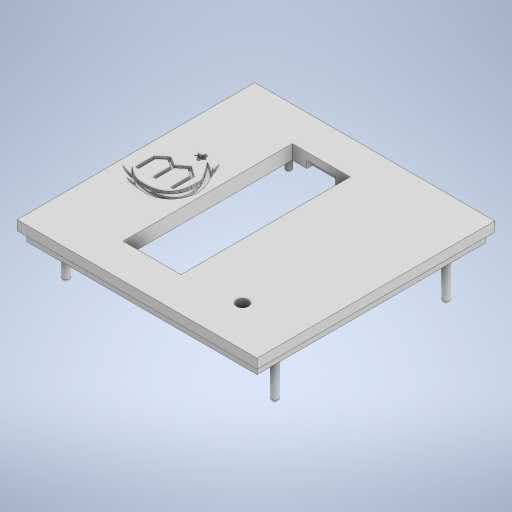
# Autodesk Inventor part: base_frontal_esp
Saved by Autodesk Inventor 2023 (Build 270158000, 158)
## iProperties
Created: 2022-11-29
Part Number: base_frontal_esp
Material: Genérico
Document SubType Name: Modeling
Designer: Inteli
Density: 1 g/cm^3
Appearance: Padrão
Author: Inteli
## iProperties of the stored document base_frontal_esp_3DPrint.ipt
Created: 2022-11-29
Part Number: base_frontal_esp_3DPrint
Material: Genérico
Document SubType Name: Modeling
Designer: Inteli
Density: 1 g/cm^3
Appearance: Padrão
Author: Inteli
Autodesk Inventor part; units mm, degrees
ref_plane "YZ Plane" through (0, 0, 0) normal (1, 0, 0) x (0, 1, 0)
ref_plane "XZ Plane" through (0, 0, 0) normal (0, 1, 0) x (-1, 0, 0)
ref_plane "XY Plane" through (0, 0, 0) normal (0, 0, 1) x (1, 0, 0)
sketch "Esboço1" plane through (0, 0, 0) normal (0, 1, 0) x (-1, 0, 0)
  line L0 (50.5, 50) -> (-50.5, 50)
  line L1 (-50.5, 50) -> (-50.5, -50)
  line L2 (-50.5, -50) -> (50.5, -50)
  line L3 (50.5, -50) -> (50.5, 50)
  line L4 (50.5, 50) -> (-50.5, -50) construction
  line L5 (-50.5, 50) -> (50.5, -50) construction
  line L6 (20.2995, 35.575) -> (-4.0005, 35.575)
  line L7 (-4.0005, 35.575) -> (-4.0005, -35.575)
  line L8 (-4.0005, -35.575) -> (20.2995, -35.575)
  line L9 (20.2995, -35.575) -> (20.2995, 35.575)
  line L10 (20.2995, 35.575) -> (-4.0005, -35.575) construction
  line L11 (-4.0005, 35.575) -> (20.2995, -35.575) construction
  line L12 (44.809, 5.8351) -> (43.5847, 5.8351)
  line L13 (43.5847, 5.8351) -> (43.5847, -1.2807)
  line L14 (44.809, -1.7713) -> (44.809, 5.8351)
  line L15 (37.4674, -1.5814) -> (37.4674, 5.8351)
  line L16 (36.2814, 5.8351) -> (36.3184, -1.9609)
  line L17 (37.4674, 5.8351) -> (36.2814, 5.8351)
  arc A0 (45.6383, 6.4318) -> (42.5276, 9.5405) centre (27.0068, -9.1007) ccw
  arc A1 (45.6383, 6.4318) -> (40.7813, 9.7169) centre (35.3189, -3.5922) ccw
  arc A2 (48.2046, 8.0198) -> (42.5276, 9.5405) centre (39.1563, -14.4019) ccw
  arc A3 (48.2046, 8.0198) -> (40.2854, 11.1296) centre (34.1591, -16.1096) ccw
  arc A4 (40.7813, 9.7169) -> (36.9942, 10.6964) centre (35.3189, -3.5922) ccw
  arc A5 (42.5276, 9.5405) -> (40.2854, 11.1296) centre (31.511, -3.6276) ccw
  arc A6 (42.5276, 9.5405) -> (39.5218, 11.5577) centre (31.511, -3.6276) ccw
  arc A7 (42.6579, 11.5577) -> (38.6679, 12.02) centre (38.9758, -2.7706) ccw
  arc A8 (42.6579, 11.5577) -> (39.3141, 12.7524) centre (36.6829, 0.1114) ccw
  arc A9 (39.5218, 11.5577) -> (37.8822, 12.3788) centre (32.6692, -0.0774) ccw
  arc A10 (32.6917, 13.3458) -> (28.802, 12.3788) centre (32.9881, 3.847) ccw
  arc A11 (32.9881, 10.9892) -> (31.7772, 10.4136) centre (38.1916, -1.5183) ccw
  arc A12 (28.802, 12.3788) -> (27.4641, 11.6847) centre (32.6917, 3.2455) ccw
  arc A13 (31.7772, 10.4136) -> (30.4336, 9.6603) centre (40.3851, -6.5145) ccw
  arc A14 (32.6139, 10.9611) -> (29.2079, 10.2542) centre (33.9158, -3.8703) ccw
  arc A15 (32.8836, 9.8314) -> (30.7097, 9.0348) centre (35.8636, -1.665) ccw
  arc A16 (27.4641, 11.6847) -> (26.2813, 10.8254) centre (32.6917, 3.2455) ccw
  arc A17 (29.2079, 10.2542) -> (27.3406, 9.3519) centre (31.9412, 2.2141) ccw
  arc A18 (29.5501, 9.0348) -> (28.6058, 8.2482) centre (39.1969, -3.5073) ccw
  arc A19 (26.2813, 10.8254) -> (24.8245, 9.2999) centre (32.6917, 3.2455) ccw
  arc A20 (30.7097, 9.0348) -> (29.0216, 7.805) centre (34.0907, 2.6203) ccw
  arc A21 (27.3406, 9.3519) -> (25.7439, 8.0198) centre (31.9412, 2.2141) ccw
  arc A22 (28.6058, 8.2482) -> (27.662, 7.2379) centre (33.3062, 2.9113) ccw
  arc A23 (24.8245, 9.2999) -> (23.5927, 7.4677) centre (38.9166, -1.505) ccw
  arc A24 (30.4336, 9.6603) -> (29.5501, 9.0348) centre (32.8777, 5.2714) ccw
  arc A25 (24.7648, 6.4318) -> (24.4302, 5.4014) centre (28.6882, 4.5883) ccw
  arc A26 (25.7439, 8.0198) -> (24.7648, 6.4318) centre (32.6186, 2.6854) ccw
  arc A27 (23.5927, 7.4677) -> (22.4449, 3.8607) centre (35.0612, 1.8321) ccw
  arc A28 (26.6056, 5.7739) -> (25.8372, 4.2176) centre (36.8949, -0.274) ccw
  arc A29 (25.8372, 4.2176) -> (25.1763, 1.9892) centre (36.8949, -0.274) ccw
  arc A30 (24.4302, 5.4014) -> (24.3636, 1.8425) centre (33.2592, 3.4561) ccw
  arc A31 (27.0068, 4.8466) -> (26.3681, 2.5448) centre (34.7317, 1.4636) ccw
  arc A32 (22.4449, 3.8607) -> (22.3296, 1.6755) centre (31.1835, 2.304) ccw
  arc A33 (26.3681, 2.5448) -> (26.168, 1.1642) centre (413.7374, -54.3143) ccw
  line L18 (29.975, 5.8351) -> (28.8297, 5.8351)
  arc A34 (22.3296, 1.6755) -> (23.1987, -2.3386) centre (36.0492, 2.5448) ccw
  arc A35 (25.1763, 1.9892) -> (24.9935, -0.598) centre (35.3122, -0.0273) ccw
  arc A36 (26.168, 1.1642) -> (26.0888, -0.901) centre (41.6964, -0.4656) ccw
  arc A37 (24.3636, 1.8425) -> (25.65, -2.2141) centre (40.1319, 4.6107) ccw
  arc A38 (26.0888, -0.901) -> (26.168, -3.3028) centre (40.7425, -1.6198) ccw
  line L19 (28.8297, 5.8351) -> (28.8297, -2.8363)
  line L20 (29.975, -2.2568) -> (29.975, 5.8351)
  line L21 (33.2053, -4.5224) -> (29.975, -2.2568)
  line L22 (28.8297, -2.8363) -> (33.2418, -6.0041)
  line L23 (36.3184, -1.9609) -> (33.2053, -4.5224)
  line L24 (40.8957, -3.6276) -> (37.4674, -1.5814)
  line L25 (33.2418, -6.0041) -> (37.1716, -2.7706)
  line L26 (37.1716, -2.7706) -> (41.0273, -5.0718)
  arc A39 (27.662, 7.2379) -> (26.6056, 5.7739) centre (37.4265, -0.9211) ccw
  arc A40 (29.0216, 7.805) -> (27.0068, 4.8466) centre (34.5802, 1.8542) ccw
  arc A41 (25.65, -2.2141) -> (27.7622, -5.9921) centre (47.4025, 7.4677) ccw
  arc A42 (24.9935, -5.6255) -> (26.0942, -6.9357) centre (36.0492, 2.5448) ccw
  arc A43 (24.9935, -5.6255) -> (25.4758, -7.1596) centre (38.388, -2.2568) ccw
  arc A44 (24.4302, -4.8024) -> (26.8873, -7.7042) centre (36.0492, 2.5448) ccw
  arc A45 (23.1987, -2.3386) -> (24.4302, -4.8024) centre (36.0492, 2.5448) ccw
  line L27 (43.5847, -1.2807) -> (40.8957, -3.6276)
  line L28 (41.0273, -5.0718) -> (44.809, -1.7713)
  line L29 (34.2937, -11.1823) -> (34.0945, -11.0661)
  line L30 (33.8991, -11.0325) -> (33.7636, -10.9072)
  line L31 (33.3989, -11.5321) -> (33.7389, -12.1961)
  line L32 (33.7389, -12.1961) -> (33.9199, -12.0962)
  line L33 (33.5923, -12.4562) -> (34.3671, -12.0313)
  line L34 (33.9199, -12.0962) -> (33.608, -11.5313)
  line L35 (33.5136, -10.9851) -> (32.8806, -11.5321)
  line L36 (33.6313, -10.6456) -> (32.6918, -11.5321)
  line L37 (33.1875, -11.5438) -> (33.5136, -10.9851)
  line L38 (33.8225, -11.5321) -> (34.0691, -12.0138)
  line L39 (34.0691, -12.0138) -> (34.2937, -11.8898)
  line L40 (33.7636, -10.9072) -> (33.3989, -11.5321)
  line L41 (33.608, -11.5313) -> (33.8991, -11.0325)
  line L42 (34.0945, -11.0661) -> (33.8225, -11.5321)
  line L43 (34.3671, -11.0482) -> (33.6313, -10.6456)
  line L44 (33.5136, -10.0703) -> (34.3671, -11.0482)
  line L45 (34.2937, -11.1823) -> (34.2937, -11.8898)
  line L46 (32.8806, -11.5321) -> (33.4944, -12.0996)
  line L47 (32.6918, -11.5321) -> (33.5923, -12.4562)
  line L48 (33.4944, -12.0996) -> (33.1875, -11.5438)
  arc A46 (25.4758, -7.1596) -> (26.168, -8.8375) centre (37.6572, -3.116) ccw
  arc A47 (26.0942, -6.9357) -> (27.0629, -8.5615) centre (38.5577, -0.6105) ccw
  arc A48 (27.0629, -8.5615) -> (27.4344, -9.9972) centre (63.4878, 0.0976) ccw
  arc A49 (27.0629, -8.5615) -> (28.2466, -10.17) centre (40.1173, -0.1951) ccw
  arc A50 (26.8873, -7.7042) -> (28.2466, -10.17) centre (61.1895, 9.5979) ccw
  arc A51 (27.4344, -9.9972) -> (27.7155, -11.1094) centre (75.5076, 1.5619) ccw
  arc A52 (26.8687, -10.2938) -> (27.4238, -11.3917) centre (91.8054, 21.8477) ccw
  arc A53 (27.7622, -5.9921) -> (31.3672, -10.9259) centre (68.3902, 19.9095) ccw
  arc A54 (26.8873, -7.7042) -> (31.3672, -10.9259) centre (41.3631, 7.6994) ccw
  arc A55 (27.7155, -11.1094) -> (28.1199, -12.5465) centre (75.5076, 1.5619) ccw
  arc A56 (27.4238, -11.3917) -> (28.1199, -12.5465) centre (38.8613, -5.2849) ccw
  arc A57 (26.168, -8.8375) -> (26.8687, -10.2938) centre (91.8054, 21.8477) ccw
  line L49 (34.8442, -10.3512) -> (34.6787, -9.7074)
  line L50 (34.6787, -9.7074) -> (33.9642, -9.5676)
  line L51 (34.8442, -10.8775) -> (34.8442, -10.3512)
  line L52 (33.9642, -9.5676) -> (33.5136, -10.0703)
  line L53 (34.6829, -11.4101) -> (34.8442, -10.8775)
  line L54 (34.3671, -11.0482) -> (34.6829, -11.4101)
  line L55 (34.6829, -11.6897) -> (34.8442, -12.2373)
  line L56 (34.3671, -12.0313) -> (34.6829, -11.6897)
  line L57 (34.8442, -12.2373) -> (35.1652, -12.4348)
  arc A58 (39.9353, 10.0335) -> (35.0612, 10.1842) centre (36.8756, -10.0261) ccw
  arc A59 (35.0612, 10.1842) -> (32.8836, 9.8314) centre (35.8636, -1.665) ccw
  arc A60 (36.9942, 10.6964) -> (32.6139, 10.9611) centre (33.9158, -3.8703) ccw
  arc A61 (37.8822, 12.3788) -> (35.3189, 13.1632) centre (32.6692, -0.0774) ccw
  arc A62 (35.3189, 13.1632) -> (32.6917, 13.3458) centre (33.3374, 3.6492) ccw
  arc A63 (39.3141, 12.7524) -> (34.7317, 13.2668) centre (35.1345, -3.8139) ccw
  line L58 (34.8798, -12.783) -> (34.8442, -12.2373)
  line L59 (34.3671, -12.0313) -> (33.4944, -12.975)
  line L60 (33.9307, -13.475) -> (34.6371, -13.3962)
  line L61 (33.4944, -12.975) -> (33.9307, -13.475)
  line L62 (34.6371, -13.3962) -> (34.8798, -12.783)
  line L63 (35.1652, -12.4348) -> (35.9116, -11.9781)
  line L64 (35.1345, -10.6456) -> (34.8442, -10.8775)
  arc A64 (36.566, -12.5465) -> (36.62, -12.3703) centre (36.3795, -12.3929) ccw
  arc A65 (36.566, -12.5465) -> (35.9116, -11.8619) centre (35.6269, -12.789) ccw
  line L65 (35.9116, -11.9781) -> (35.9116, -11.1094)
  arc A66 (36.62, -12.3703) -> (35.9116, -11.6487) centre (35.5381, -12.7239) ccw
  line L66 (35.9116, -11.1094) -> (35.1345, -10.6456)
  arc A67 (35.9116, -11.3917) -> (36.62, -10.6875) centre (35.6092, -10.3791) ccw
  arc A68 (35.9116, -11.2016) -> (36.5905, -10.5013) centre (35.3642, -9.9917) ccw
  arc A69 (36.62, -10.6875) -> (36.5905, -10.5013) centre (36.2493, -10.6509) ccw
  point P0 (0, 0)
  point P1 (28.6058, 8.2482)
  dimension "d0" = 101
  dimension "d1" = 100
  dimension "d2" = 24.3
  dimension "d3" = 71.15
  constraints: 165 point on circle, 134 end point, 70 centre point, 16 parallel, 12 point on line, 10 concentric, 8 perpendicular, 3 horizontal, 3 vertical, 2 midpoint
  measures "d0" distance of L2.end L1.end
  measures "d1" distance of L1.end L0.end
  measures "d2" distance of L8.end L7.end
  measures "d3" distance of L7.end L6.end
extrude "Base" add sketch "Esboço1" against normal blind 8 contours L3 L2 L1 L0 | L14 L28 L26 L25 L22 L19 L18 L20 L21 L23 L16 L17 L15 L24 L27 L13 L12 | A1 A4 A60 A14 A17 A21 A26 A25 A30 A37 A41 A53 A54 A44 A42 A45 A34 A32 A27 A23 A19 A16 A12 A10 A62 A61 A9 A6 A5 A0 | A5 A3 A2 | A58 A59 A15 A20 A40 A31 A33 A36 A38 A41 A37 A35 A29 A28 A39 A22 A18 A24 A13 A11 A60 A4 | A9 A61 A62 A63 A8 A7 | A11 A13 A24 A18 A22 A39 A28 A29 A35 A37 A30 A25 A26 A21 A17 A14 A60 | A50 A49 A47 A44 | A47 A48 A51 A55 A56 A52 A57 A46 A43 A42 | L45 L39 L38 L42 L29 | L41 L34 L32 L31 L40 L30 | L47 L36 L43 L54 L53 L64 L66 L65 L63 L57 L55 L56 L33 | L56 L55 L58 L62 L60 L61 L59 | L44 L52 L50 L49 L51 L53 L54 | L65 A66 A64 A65 | L65 A68 A69 A67 | L37 L48 L46 L35
sketch "Esboço4" plane through (0, -8, 0) normal (0, -1, 0) x (1, 0, 0)
  line L0 (-48, 40) -> (-48, -40) projected
  line L1 (48, -40) -> (48, 40) projected
  circle A0 centre (-44, -36) radius 1.5
  circle A1 centre (-44, 36) radius 1.5
  circle A2 centre (44, 36) radius 1.5
  circle A3 centre (44, -36) radius 1.5
  line L2 (-50.5, 50) -> (-50.5, -50) projected
  line L3 (50.5, 50) -> (-50.5, 50) projected
  point P0 (0, 0)
  dimension "d21" = 3
  dimension "d22" = 3
  dimension "d23" = 3
  dimension "d24" = 3
  dimension "d82" = 6.5
  dimension "d83" = 14
  constraints: 4 centre point
  measures "d21" diameter of A0
  measures "d22" diameter of A1
  measures "d23" diameter of A2
  measures "d24" diameter of A3
  measures "d82" distance from line of L2 A1.centre
  measures "d83" distance from line of L3 A1.centre
extrude "Pinos_encaixe" add sketch "Esboço4" along normal blind 18
fillet "Arredondamento_pino" radius 1.5 4 edges at (-45.5, -26, -36) (-45.5, -26, 36) (42.5, -26, 36) (42.5, -26, -36)
extrude "Logo Iobee C.1" cut sketch "Esboço1" against normal blind 1.5 contours L14 L28 L26 L25 L22 L19 L18 L20 L21 L23 L16 L17 L15 L24 L27 L13 L12 | A1 A4 A60 A14 A17 A21 A26 A25 A30 A37 A41 A53 A54 A44 A42 A45 A34 A32 A27 A23 A19 A16 A12 A10 A62 A61 A9 A6 A5 A0 | L45 L39 L38 L42 L29 | L41 L34 L32 L31 L40 L30 | L47 L36 L43 L54 L53 L64 L66 L65 L63 L57 L55 L56 L33 | L56 L55 L58 L62 L60 L61 L59 | L44 L52 L50 L49 L51 L53 L54 | L65 A66 A64 A65 | L65 A68 A69 A67 | L37 L48 L46 L35
extrude "Logo Iobee C.2" cut sketch "Esboço1" against normal blind 1 contours A5 A3 A2 | A58 A59 A15 A20 A40 A31 A33 A36 A38 A41 A37 A35 A29 A28 A39 A22 A18 A24 A13 A11 A60 A4 | A47 A48 A51 A55 A56 A52 A57 A46 A43 A42
extrude "Logo Iobee C.3" cut sketch "Esboço1" against normal blind 0.5 contours A9 A61 A62 A63 A8 A7 | A11 A13 A24 A18 A22 A39 A28 A29 A35 A37 A30 A25 A26 A21 A17 A14 A60 | A50 A49 A47 A44
sketch "Esboço_ESP32" plane through (0, -8, 0) normal (0, -1, 0) x (1, 0, 0)
  line L0 (13.3, -50) -> (41.3, -50)
  line L1 (41.3, -50) -> (41.3, 10)
  line L2 (41.3, 10) -> (13.3, 10)
  line L3 (13.3, 10) -> (13.3, -50)
  line L4 (17.8, 10) -> (36.8, 10)
  line L5 (36.8, 10) -> (36.8, 18)
  line L6 (36.8, 18) -> (17.8, 18)
  line L7 (17.8, 18) -> (17.8, 10)
  line L8 (-50.5, -50) -> (50.5, -50) projected
  line L9 (50.5, -50) -> (50.5, 50) projected
  point P0 (0, 0)
  point P1 (13.3133, -50)
  dimension "d34" = 28
  dimension "d35" = 60
  dimension "d36" = 19
  dimension "d37" = 8
  dimension "d38" = 4.5
  dimension "d84" = 9.2
  constraints: 16 end point, 4 parallel, 2 horizontal, 2 perpendicular, 2 point on line
  measures "d34" distance of L2.end L1.end
  measures "d35" distance of L1.end L0.end
  measures "d36" distance of L6.end L5.end
  measures "d37" distance of L5.end L4.end
  measures "d38" distance between parallel lines of L1 L5
  measures "d84" distance between parallel lines of L9 L1
extrude "ESP32_alocar" cut sketch "Esboço_ESP32" against normal blind 5 contours L3 L2 L1 L0
extrude "ESP32_Wi-Fi" cut sketch "Esboço_ESP32" against normal blind 3 contours L7 L6 L5 L2
sketch "Esboço_LCD_dentro" plane through (0, -8, 0) normal (0, -1, 0) x (1, 0, 0)
  line L0 (-20.2995, -35.575) -> (4.0005, -35.575) projected
  line L1 (4.0005, -35.575) -> (4.0005, 35.575) projected
  line L2 (-26.1745, -39.95) -> (9.8755, -39.95)
  line L3 (9.8755, -39.95) -> (9.8755, 39.95)
  line L4 (9.8755, 39.95) -> (-26.1745, 39.95)
  line L5 (-26.1745, 39.95) -> (-26.1745, -39.95)
  line L6 (-26.1745, -39.95) -> (9.8755, 39.95) construction
  line L7 (9.8755, -39.95) -> (-26.1745, 39.95) construction
  point P0 (0, 0)
  point P1 (-8.1495, 0)
  dimension "d44" = 36.05
  dimension "d45" = 79.9
  constraints: 12 end point, 2 midpoint, 2 parallel, 1 horizontal, 1 perpendicular
  measures "d44" distance of L4.end L3.end
  measures "d45" distance of L3.end L2.end
extrude "LCD_Dentro" cut sketch "Esboço_LCD_dentro" against normal blind 2
sketch "Esboço7" plane through (0, -6, 0) normal (0, -1, 0) x (1, 0, 0)
  line L0 (-20.2995, 35.575) -> (-20.2995, -35.575) projected
  line L1 (4.0005, 35.575) -> (-20.2995, 35.575) projected
  line L2 (-20.2995, -35.575) -> (4.0005, 35.575)
  line L3 (4.0005, -35.575) -> (4.0005, 35.575) projected
  line L4 (4.0005, -35.575) -> (-20.2995, 35.575)
  line L5 (-20.2995, -35.575) -> (4.0005, -35.575) projected
  line L6 (-8.1495, -35.575) -> (-14.1495, -35.575)
  line L7 (-14.1495, -35.575) -> (-14.1495, -39.95)
  line L8 (9.8755, -39.95) -> (-26.1745, -39.95) projected
  line L9 (-14.1495, -39.95) -> (-2.1495, -39.95)
  line L10 (-2.1495, -39.95) -> (-2.1495, -35.575)
  line L11 (-2.1495, -35.575) -> (-8.1495, -35.575)
  line L12 (-26.1745, -39.95) -> (-26.1745, 39.95) projected
  line L13 (-26.1745, -6.25) -> (-22.1745, -6.25)
  line L14 (-22.1745, -6.25) -> (-22.1745, 33.75)
  line L15 (-22.1745, 33.75) -> (-26.1745, 33.75)
  line L16 (-26.1745, 33.75) -> (-26.1745, -6.25)
  line L17 (-26.1745, 39.95) -> (9.8755, 39.95) projected
  point P0 (0, 0)
  dimension "d54" = 4
  dimension "d55" = 40
  dimension "d56" = 6.2
  constraints: 22 end point, 4 point on line, 2 parallel, 2 perpendicular, 1 horizontal, 1 midpoint, 1 vertical
  measures "d54" distance of L15.end L14.end
  measures "d55" distance of L14.end L13.end
  measures "d56" distance between parallel lines of L17 L15
extrude "Chaveta_LCD" cut sketch "Esboço7" against normal blind 3 contours L5 L10 L8 L7
extrude "LCD Pinos" cut sketch "Esboço7" against normal blind 4 contours L12 L15 L14 L13
sketch "Esboço8" plane through (0, -8, 0) normal (0, -1, 0) x (1, 0, 0)
  line L0 (50.5, -50) -> (50.4652, -50)
  line L1 (-50.5, -50) -> (-50.5, 50) projected
  line L2 (-50.5, -50) -> (50.5, -50)
  line L3 (50.5, -50) -> (50.5, 50)
  line L4 (50.5, 50) -> (-50.5, 50)
  line L5 (-50.5, 50) -> (-50.5, -50)
  line L6 (-48.5, 48) -> (48.5, 48)
  line L7 (48.5, 48) -> (48.5, -48)
  line L8 (48.5, -48) -> (-48.5, -48)
  line L9 (-48.5, -48) -> (-48.5, 48)
  point P0 (0, 0)
  point P1 (-50.5, 50)
  point P2 (50.5, -50)
  dimension "d80" = 96
  dimension "d81" = 97
  constraints: 18 end point, 4 parallel, 2 perpendicular, 1 horizontal, 3 other
  measures "d80" distance of L6.end L7.end
  measures "d81" distance of L6.start L6.end
extrude "Rasgo de Encaixe" cut sketch "Esboço8" against normal blind 4
sketch "Esboço9" plane through (0, -8, 0) normal (0, -1, 0) x (1, 0, 0)
  point P0 (0, 0)
sketch "Esboço10" plane through (0, -6, 0) normal (0, -1, 0) x (1, 0, 0)
  line L0 (-26.1745, 39.95) -> (9.8755, 39.95) projected
  circle A0 centre (-24.1745, -37.95) radius 1.25
  circle A1 centre (-24.1745, 37.95) radius 1.25
  circle A2 centre (7.8755, 37.95) radius 1.25
  circle A3 centre (7.8755, -37.95) radius 1.25
  line L1 (9.8755, 39.95) -> (9.8755, -39.95) projected
  point P0 (0, 0)
  point P1 (-26.1745, -39.95)
  dimension "d68" = 2.5
  dimension "d69" = 2.5
  dimension "d70" = 2.5
  dimension "d71" = 2.5
  dimension "d73" = 75.9
  dimension "d86" = 32.05
  dimension "d88" = 2
  constraints: 4 centre point
  measures "d68" diameter of A0
  measures "d69" diameter of A1
  measures "d70" diameter of A2
  measures "d71" diameter of A3
  measures "d73" distance of A2.centre A3.centre
  measures "d86" distance of A2.centre A1.centre
  measures "d88" distance from line of L1 A3.centre
extrude "Pinos Guia LCD" add sketch "Esboço10" along normal blind 7
fillet "Arredondamento2" radius 1 4 edges at (-25.4245, -13, -37.95) (-25.4245, -13, 37.95) (6.6255, -13, 37.95) (6.6255, -13, -37.95)
sketch "Esboço11" plane through (0, -8, 0) normal (0, -1, 0) x (1, 0, 0)
  circle A0 centre (27.3133, 33) radius 2.5
  line L0 (17.8, 18) -> (36.8, 18) projected
  line L1 (48.5, 48) -> (-48.5, 48) projected
  point P0 (0, 0)
  dimension "d77" = 5
  constraints: 1 centre point
  measures "d77" diameter of A0
extrude "Furo Led" cut sketch "Esboço11" against normal through all
